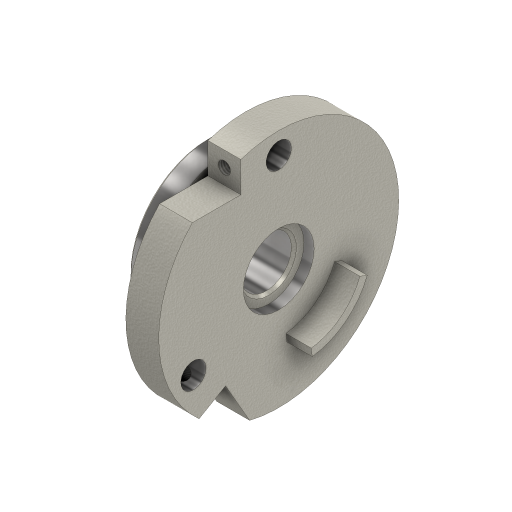
# Autodesk Inventor part: Part032.Front support
Saved by Autodesk Inventor 2023.2 (Build 272271030, 271C)
## iProperties
Created: 2023-11-08
Part Number: Part032.Front support
Material: Steel, Cast
Document SubType Name: Modeling
Designer: User
Mass: 934.407 g
Surface Area: 245.939 cm^2
Volume: 119.033 cm^3
Density: 7.85 g/cm^3
Appearance: Steel - Cast
Author: User
Autodesk Inventor part; units mm, degrees
note: some values were not read from the file. Chosen so that the rebuilt part matches the saved one: direction of "Hole2".
ref_plane "YZ Plane" through (0, 0, 0) normal (1, 0, 0) x (0, 1, 0)
ref_plane "XZ Plane" through (0, 0, 0) normal (0, 1, 0) x (-1, 0, 0)
ref_plane "XY Plane" through (0, 0, 0) normal (0, 0, 1) x (1, 0, 0)
sketch "Sketch1" plane through (0, 0, 0) normal (0, 0, 1) x (1, 0, 0)
  line L0 (0, 0) -> (0, 10) construction
  line L1 (0, 31.5) -> (10, 31.5)
  line L2 (10, 31.5) -> (10, 27)
  line L3 (10, 27) -> (15, 27)
  line L4 (15, 27) -> (15, 47.5)
  line L5 (15, 47.5) -> (28, 47.5)
  line L6 (28, 47.5) -> (28, 14)
  line L7 (28, 0) -> (0, 0)
  line L8 (0, 10) -> (24, 10)
  line L9 (24, 10) -> (24, 14)
  line L10 (24, 14) -> (28, 14)
  line L11 (0, 10) -> (0, 31.5)
  line L12 (28, 14) -> (28, 0) construction
  dimension "d0" = 95
  dimension "d1" = 54
  dimension "d2" = 63
  dimension "d3" = 20
  dimension "d4" = 28
  dimension "d5" = 4
  dimension "d6" = 28
  dimension "d7" = 13
  dimension "d8" = 10
  constraints: 26 end point, 10 perpendicular, 3 vertical, 2 horizontal
  measures "d0" diameter of L5 L7
  measures "d1" diameter of L3 L7
  measures "d2" diameter of L1 L7
  measures "d3" diameter of L8 L7
  measures "d4" diameter of L10 L7
  measures "d5" distance of L9.end L6.end
  measures "d6" distance between parallel lines of L6 L11
  measures "d7" distance of L4.end L5.end
  measures "d8" distance of L1.start L1.end
revolve "Revolution1" add sketch "Sketch1" angle 360 about axis through (28, 0, 0) along (-1, 0, 0)
chamfer "Chamfer1" distance 1 angle 45 4 edges at (24, -10, 0) (0, -10, 0) (10, -31.5, 0) (0, -31.5, 0)
sketch "Sketch2" plane through (28, 0, 0) normal (1, 0, 0) x (0, 0, -1)
  circle A0 centre (0, 0) radius 47.5 projected
  circle A1 centre (0, 0) radius 14 projected
  arc A2 (3.2661, -26.6002) -> (25.02, -9.6043) centre (0, 0) ccw
  arc A3 (2.8883, -23.5233) -> (22.1259, -8.4933) centre (0, 0) ccw
  line L0 (2.8883, -23.5233) -> (3.2661, -26.6002)
  line L1 (22.1259, -8.4933) -> (25.02, -9.6043)
  line L2 (0, 0) -> (0, -47.5)
  dimension "d13" = 7
  dimension "d14" = 62
  dimension "d15" = 23.7
  dimension "d16" = 26.8
  constraints: 6 end point, 4 point on circle, 2 centre point, 2 coincident, 2 point on line, 1 vertical, 1 vertical alignment, 1 other
  measures "d13" angle of L0 L2
  measures "d14" angle of L1 L0
  measures "d15" radius of A3
  measures "d16" radius of A2
extrude "Extrusion1" add sketch "Sketch2" along normal blind 10 contours L0 A3 L1 A2
sketch "Sketch3" plane through (28, 0, 0) normal (1, 0, 0) x (0, 0, -1)
  arc A0 (2.8883, -23.5233) -> (22.1259, -8.4933) centre (0, 0) ccw projected
  circle A1 centre (0, 0) radius 47.5 projected
  line L0 (-34.165, 33) -> (-15, 33)
  line L1 (-15, 33) -> (-15, 45.0694)
  dimension "d19" = 33
  dimension "d20" = 15
  constraints: 4 end point, 2 point on circle, 1 horizontal, 1 perpendicular
  measures "d19" distance from line of A0.centre L0
  measures "d20" distance from line of A0.centre L1
extrude "Extrusion2" cut sketch "Sketch3" against normal through all contours L1 L0 A1 picked at (-25.8726, 34.6785)
sketch "Sketch4" plane through (28, 33, 15) normal (1, 0, 0) x (0, 0, -1)
  circle A0 centre (15, -33) radius 14 projected
  line L0 (0, 0) -> (-19.165, 0) projected
  point P0 (15, 6)
  dimension "d23" = 6
  constraints: 1 vertical alignment
  measures "d23" distance from line of L0 point (15, 6)
hole "Hole1" at (28, 39, 0) direction (-1, 0, 0) diameter 10 end through all
sketch "Sketch5" plane through (28, 33, 15) normal (0, 0, 1) x (1, 0, 0)
  line L0 (0, 0) -> (-13, 0) projected
  line L1 (-13, 12.0694) -> (0, 12.0694) projected
  point P0 (-28, -33)
  point P1 (-6.5, 6)
  point P2 (-6.5, 12.0694)
  dimension "d31" = 6
  constraints: 1 midpoint, 1 vertical alignment
  measures "d31" distance from line of L0 point (-6.5, 6)
hole "Hole2" at (21.5, 39, 15) direction (0, 0, -1) diameter 4.917 end up to surface thread size "M6x1" class "6H" standard "ISO Metric profile"
pattern_circular "Circular Pattern1" count 2 over 120 about axis through (21.5, 0, 0) along (1, 0, 0) of "Hole2", "Hole1", "Extrusion2"
sketch "Sketch6" plane through (24, 0, 0) normal (1, 0, 0) x (0, 0, -1)
  circle A0 centre (0, 0) radius 14 projected
  line L0 (-3, 0) -> (3, 0)
  line L1 (3, 0) -> (3, 12.3)
  line L2 (3, 12.3) -> (-3, 12.3)
  line L3 (-3, 12.3) -> (-3, 0)
  dimension "d42" = 12.3
  dimension "d43" = 6
  constraints: 8 end point, 2 parallel, 1 coincident, 1 horizontal, 1 midpoint, 1 perpendicular
  measures "d42" distance between parallel lines of L0 L2
  measures "d43" distance between parallel lines of L1 L3
extrude "Extrusion3" cut sketch "Sketch6" against normal through all contours L3 L2 L1 L0
body "Solid1"
